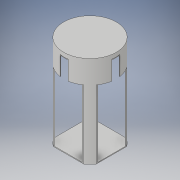
# Autodesk Inventor part: Hull
Saved by Autodesk Inventor 2018 (Build 220112000, 112)
## iProperties
Created: 2017-12-27
Part Number: Hull
Material: Generic
Document SubType Name: Modeling
Designer: Suchanek
Density: 1 g/cm^3
Appearance: Default
Author: Suchanek
Autodesk Inventor part; units mm, degrees
ref_plane "YZ Plane" through (0, 0, 0) normal (1, 0, 0) x (0, 1, 0)
ref_plane "XZ Plane" through (0, 0, 0) normal (0, 1, 0) x (-1, 0, 0)
ref_plane "XY Plane" through (0, 0, 0) normal (0, 0, 1) x (1, 0, 0)
sketch "Sketch1" plane through (0, 0, 0) normal (0, 0, 1) x (1, 0, 0)
  line L0 (0, 0) -> (33, 0)
  line L1 (33, 0) -> (33, 1)
  line L2 (33, 1) -> (0, 1)
  line L3 (0, 1) -> (0, 0)
  line L4 (33, 0) -> (32, 0)
  line L5 (32, 0) -> (32, 115)
  line L6 (32, 115) -> (33, 115)
  line L7 (33, 115) -> (33, 0)
  line L8 (33, 115) -> (0, 115)
  line L9 (0, 115) -> (0, 114)
  line L10 (0, 114) -> (33, 114)
  line L11 (33, 114) -> (33, 115)
  line L12 (0, 114) -> (0, 1)
  line L13 (-5, 105) -> (5, 105)
  line L14 (5, 105) -> (5, 5)
  line L15 (5, 5) -> (-5, 5)
  line L16 (-5, 5) -> (-5, 105)
  dimension "d0" = 33
  dimension "d1" = 1
  dimension "d2" = 1
  dimension "d3" = 115
  dimension "d4" = 33
  dimension "d5" = 1
  dimension "d6" = 10
  dimension "d7" = 100
  dimension "d8" = 4
  constraints: 34 end point, 8 parallel, 4 perpendicular, 3 horizontal, 1 other
  measures "d0" distance of L2.end L1.end
  measures "d1" distance of L1.end L0.end
  measures "d2" distance of L5.end L6.end
  measures "d3" distance of L4.end L5.end
  measures "d4" distance of L10.end L9.end
  measures "d5" distance of L9.end L8.end
  measures "d6" distance of L14.end L15.end
  measures "d7" distance of L15.end L13.start
  measures "d8" distance from line of L1.end L15
sketch "Sketch2" plane through (0, 0, 0) normal (1, 0, 0) x (0, 1, 0)
  line L0 (110, 5) -> (5, 5)
  line L1 (5, 5) -> (5, -5)
  line L2 (5, -5) -> (110, -5)
  line L3 (110, -5) -> (110, 5)
  line L4 (0, 0) -> (0, -10)
  line L5 (0, 0) -> (115, 0)
  dimension "d9" = 10
  dimension "d10" = 5
  dimension "d12" = 115
  dimension "d13" = 10
  dimension "d14" = 105
  constraints: 12 end point, 2 horizontal, 2 parallel, 1 perpendicular, 1 vertical, 1 other
  measures "d9" distance of L4.start L4.end
  measures "d10" distance between parallel lines of L1 L4
  measures "d12" distance of L4.start L5.end
  measures "d13" distance between parallel lines of L0 L2
  measures "d14" distance of L1.end L2.end
extrude "Extrusion1" add sketch "Sketch2" along normal mid plane 10
revolve "Revolution1" add sketch "Sketch1" angle 360 about axis through (0, 114, 0) along (0, -1, 0) contours L3 L2 L5 L0 | L5 L2 L1 L0 | L5 L10 L7 L2 | L10 L9 L8 L5 | L5 L6 L7 L10
sketch "Sketch3" plane through (-5, 5, 5) normal (0, 0, 1) x (1, 0, 0)
  line L0 (0, 105) -> (10, 105) projected
  line L1 (10, 105) -> (10, 0) projected
  line L2 (0, 105) -> (10, 105)
  line L3 (10, 105) -> (10, 0)
  line L4 (10, 0) -> (0, 0)
  line L5 (0, 0) -> (0, 105)
  point P0 (5, -5)
  dimension "d18" = 105
  constraints: 8 end point, 2 parallel, 1 horizontal, 1 perpendicular
  measures "d18" distance of L2.end L1.end
extrude "Extrusion2" cut sketch "Sketch3" along normal mid plane 200
sketch "Sketch4" plane through (5, 0, 0) normal (1, 0, 0) x (0, 0, -1)
  line L0 (-5, 110) -> (-5, 5) projected
  line L1 (-5, 110) -> (5, 110)
  line L2 (5, 110) -> (5, 5)
  line L3 (5, 5) -> (-5, 5)
  line L4 (-5, 5) -> (-5, 110)
  point P0 (0, 0)
  dimension "d21" = 10
  constraints: 8 end point, 2 parallel, 1 horizontal, 1 perpendicular, 1 point on line
  measures "d21" distance of L2.end L3.end
extrude "Extrusion3" cut sketch "Sketch4" along normal mid plane 200
sketch "Sketch5" plane through (-32.619, 5, -5) normal (0, 0, 1) x (1, 0, 0)
  line L0 (1.0121, 105) -> (0, 105) projected
  line L1 (0, 105) -> (1, 105)
  line L2 (1, 105) -> (1, 104)
  line L3 (1, 104) -> (0, 104)
  line L4 (0, 104) -> (0, 105)
  line L5 (65.238, 105) -> (64.226, 105) projected
  line L6 (65.238, 105) -> (64.238, 105)
  line L7 (64.238, 105) -> (64.238, 104)
  line L8 (64.238, 104) -> (65.238, 104)
  line L9 (65.238, 104) -> (65.238, 105)
  point P0 (32.619, -5)
  dimension "d24" = 1
  dimension "d25" = 1
  dimension "d26" = 1
  dimension "d27" = 1
  constraints: 16 end point, 4 parallel, 2 horizontal, 2 perpendicular
  measures "d24" distance of L2.end L3.end
  measures "d25" distance of L1.end L2.end
  measures "d26" distance of L8.end L7.end
  measures "d27" distance of L7.end L6.end
extrude "Extrusion4" add sketch "Sketch5" along normal blind 10
sketch "Sketch6" plane through (5, 5, 31.607) normal (-1, 0, 0) x (0, 0, 1)
  line L0 (0, 105) -> (1.0121, 105) projected
  line L1 (1.0121, 105) -> (0.0121, 105)
  line L2 (0.0121, 105) -> (0.0121, 104)
  line L3 (0.0121, 104) -> (1.0121, 104)
  line L4 (1.0121, 104) -> (1.0121, 105)
  line L5 (-64.226, 105) -> (-63.2139, 105) projected
  line L6 (-64.226, 105) -> (-63.226, 105)
  line L7 (-63.226, 105) -> (-63.226, 104)
  line L8 (-63.226, 104) -> (-64.226, 104)
  line L9 (-64.226, 104) -> (-64.226, 105)
  point P0 (-31.607, -5)
  dimension "d30" = 1
  dimension "d31" = 1
  dimension "d32" = 1
  dimension "d33" = 1
  constraints: 16 end point, 4 parallel, 2 horizontal, 2 perpendicular
  measures "d30" distance of L3.end L2.end
  measures "d31" distance of L2.end L1.end
  measures "d32" distance of L7.end L8.end
  measures "d33" distance of L6.end L7.end
extrude "Extrusion5" add sketch "Sketch6" along normal blind 10
sketch "Sketch7" plane through (0, 1, 0) normal (0, 1, 0) x (1, 0, 0)
  line L0 (0, 0) -> (-27, 0)
  line L1 (-27, 0) -> (-27, 27)
  line L2 (-27, 27) -> (0, 27)
  line L3 (0, 27) -> (0, 0)
  line L4 (-27, 27) -> (27, 27)
  line L5 (27, 27) -> (27, 33)
  line L6 (27, 33) -> (-27, 33)
  line L7 (-27, 33) -> (-27, 27)
  line L8 (27, 27) -> (33, 27)
  line L9 (33, 27) -> (33, -27)
  line L10 (33, -27) -> (27, -27)
  line L11 (27, -27) -> (27, 27)
  line L12 (-27, 27) -> (-33, 27)
  line L13 (-33, 27) -> (-33, -27)
  line L14 (-33, -27) -> (-27, -27)
  line L15 (-27, -27) -> (-27, 27)
  line L16 (-27, -27) -> (27, -27)
  line L17 (27, -27) -> (27, -33)
  line L18 (27, -33) -> (-27, -33)
  line L19 (-27, -33) -> (-27, -27)
  dimension "d36" = 27
  dimension "d37" = 27
  dimension "d38" = 54
  dimension "d39" = 6
  dimension "d40" = 6
  dimension "d41" = 54
  dimension "d42" = 6
  dimension "d43" = 54
  dimension "d44" = 54
  dimension "d45" = 6
  constraints: 40 end point, 10 parallel, 5 horizontal, 5 perpendicular
  measures "d36" distance of L1.end L2.end
  measures "d37" distance of L0.end L1.end
  measures "d38" distance of L6.end L5.end
  measures "d39" distance of L5.end L4.end
  measures "d40" distance of L9.end L10.end
  measures "d41" distance of L8.end L9.end
  measures "d42" distance of L14.end L13.end
  measures "d43" distance of L13.end L12.end
  measures "d44" distance of L17.end L18.end
  measures "d45" distance of L16.end L17.end
extrude "Extrusion6" cut sketch "Sketch7" along normal blind 85 and the other way blind 5 contours L15 L14 L13 L12 L1 | L2 L7 L6 L5 L4 | L16 L17 L18 L19 | L8 L9 L10 L11
body "Solid1"
